Braces (Autodesk Fusion 360 design; units mm, degrees)
Autodesk Fusion 360 part; units mm, degrees
sketch "Sketch1" plane through (0, 0, 0) normal (0, 0, 1) x (1, 0, 0)
  line L0 (0, 0) -> (-170, 0)
  line L1 (-170, 0) -> (-170, 20)
  line L2 (-170, 20) -> (0, 20)
  line L3 (0, 20) -> (0, 0)
  line L4 (-140, 40) -> (-120, 40)
  line L5 (-120, 40) -> (-120, -80)
  line L6 (-120, -80) -> (-140, -80)
  line L7 (-140, -80) -> (-140, 40)
  line L8 (-66.7762, 51.8423) -> (-16.7762, 51.8423)
  line L9 (-16.7762, 51.8423) -> (-16.7762, 41.8423)
  line L10 (-16.7762, 41.8423) -> (-66.7762, 41.8423)
  line L11 (-66.7762, 41.8423) -> (-66.7762, 51.8423)
  line L12 (-66.7762, 51.8423) -> (-16.7762, 51.8423)
  line L13 (-16.7762, 51.8423) -> (-16.7762, 53.8423)
  line L14 (-16.7762, 53.8423) -> (-66.7762, 53.8423)
  line L15 (-66.7762, 53.8423) -> (-66.7762, 51.8423)
  dimension "d1" = 170
  dimension "d2" = 20
  dimension "d3" = 20
  dimension "d4" = 120
  dimension "d5" = 20
  dimension "d6" = 30
  dimension "d7" = 50
  dimension "d8" = 10
  dimension "d9" = 2
  constraint horizontal L0
  constraint vertical L1
  constraint horizontal L2
  constraint vertical L3
  constraint coincident L0.start L3.end
  constraint horizontal L4
  constraint vertical L5
  constraint horizontal L6
  constraint vertical L7
  constraint horizontal L8
  constraint vertical L9
  constraint horizontal L10
  constraint vertical L11
  constraint horizontal L12
  constraint vertical L13
  constraint horizontal L14
  constraint vertical L15
  measures "d1" distance of L0.start L0.end
  measures "d2" distance of L0.start L2.end
  measures "d3" distance of L4.start L4.end
  measures "d4" distance of L4.start L6.end
  measures "d5" distance of L2 L4
  measures "d6" distance of L1 L7
  measures "d7" distance of L8.start L8.end
  measures "d8" distance of L8.start L10.end
  measures "d9" distance of L8.start L14.end
extrude "Extrude1" add sketch "Sketch1" along normal blind 12 contours L8 L12 L13 L14 L15 makes body 1
extrude "Extrude2" add sketch "Sketch1" along normal blind 2 contours L8 L9 L10 L11 L12 bodies 1
extrude "Extrude3" add sketch "Sketch1" along normal blind 2 separate body contours L0 L2 L3 L5 | L0 L5 L6 L7 | L0 L2 L5 L7 | L0 L1 L2 L7 | L2 L4 L5 L7 makes body 2
sketch "Sketch2" plane through (0, 0, 0) normal (0, 0, 1) x (1, 0, 0)
  line L0 (-60.8582, -31.183) -> (-30.8582, -31.183)
  line L1 (-30.8582, -31.183) -> (-30.8582, -61.183)
  line L2 (-30.8582, -61.183) -> (-60.8582, -61.183)
  line L3 (-60.8582, -61.183) -> (-60.8582, -31.183)
  dimension "d16" = 30
  dimension "d17" = 30
  constraint horizontal L0
  constraint vertical L1
  constraint horizontal L2
  constraint vertical L3
  measures "d16" distance of L0.start L0.end
  measures "d17" distance of L0.start L2.end
extrude "Extrude4" add sketch "Sketch2" along normal blind 2 separate body makes body 3
sketch "Sketch3" plane through (0, 0, 0) normal (0, 0, 1) x (1, 0, 0)
  line L0 (-110.5818, 100.3288) -> (-80.5818, 100.3288)
  line L1 (-80.5818, 100.3288) -> (-80.5818, 90.3288)
  line L2 (-80.5818, 90.3288) -> (-110.5818, 90.3288)
  line L3 (-110.5818, 90.3288) -> (-110.5818, 100.3288)
  dimension "d20" = 30
  dimension "d21" = 10
  constraint horizontal L0
  constraint vertical L1
  constraint horizontal L2
  constraint vertical L3
  measures "d20" distance of L0.start L0.end
  measures "d21" distance of L0.start L2.end
extrude "Extrude5" add sketch "Sketch3" along normal blind 2 separate body makes body 4
